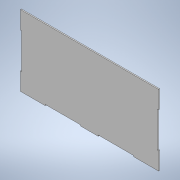
# Autodesk Inventor part: Base trasera
Saved by Autodesk Inventor 2020 (Build 240168000, 168)
## iProperties
Created: 2020-03-15
Part Number: Base trasera
Material: Genérico
Document SubType Name: Modeling
Designer: JRoCC97
Density: 1 g/cm^3
Appearance: Valor por defecto
Author: JRoCC97
Autodesk Inventor part; units mm, degrees
ref_plane "YZ Plane" through (0, 0, 0) normal (1, 0, 0) x (0, 1, 0)
ref_plane "XZ Plane" through (0, 0, 0) normal (0, 1, 0) x (-1, 0, 0)
ref_plane "XY Plane" through (0, 0, 0) normal (0, 0, 1) x (1, 0, 0)
sketch "Boceto1" plane through (0, 0, 0) normal (0, 0, 1) x (1, 0, 0)
  line L0 (0, 200) -> (390, 200)
  line L1 (70, 0) -> (70, 3)
  line L2 (70, 3) -> (170, 3)
  line L3 (170, 3) -> (170, 0)
  line L4 (220, 0) -> (220, 3)
  line L5 (220, 3) -> (320, 3)
  line L6 (320, 3) -> (320, 0)
  line L7 (70, 0) -> (0, 0)
  line L8 (390, 0) -> (320, 0)
  line L9 (220, 0) -> (170, 0)
  line L10 (0, 150) -> (3, 150)
  line L11 (3, 150) -> (3, 50)
  line L12 (3, 50) -> (0, 50)
  line L13 (0, 0) -> (0, 50)
  line L14 (0, 150) -> (0, 200)
  line L15 (390, 150) -> (387, 150)
  line L16 (387, 150) -> (387, 50)
  line L17 (387, 50) -> (390, 50)
  line L18 (390, 200) -> (390, 150)
  line L19 (390, 50) -> (390, 0)
  dimension "d7" = 100
  dimension "d9" = 100
  dimension "d10" = 200
  dimension "d11" = 3
  dimension "d17" = 3
  dimension "d18" = 100
  dimension "d20" = 50
  dimension "d23" = 390
  constraints: 40 end point, 21 perpendicular, 7 parallel, 6 collinear, 2 equal length, 2 horizontal, 1 coincident, 1 vertical
  measures "d7" distance between parallel lines of L1 L3
  measures "d9" distance of L4.end L5.end
  measures "d10" distance between parallel lines of L0 L8
  measures "d11" distance between parallel lines of L7 L2
  measures "d17" distance of L10.start L10.end
  measures "d18" distance of L10.end L11.end
  measures "d20" distance between parallel lines of L0 L10
  measures "d23" distance between parallel lines of L14 L18
extrude "Extrusión1" add sketch "Boceto1" along normal blind 3
